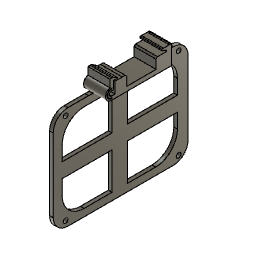
Mounting rack for editing v6 (Autodesk Fusion 360 design; units mm, degrees)
Autodesk Fusion 360 part; units mm, degrees
sketch "Sketch5" plane through (0, 0, 0) normal (1, 0, 0) x (0, 1, 0)
  line L0 (-84.5941, 0) -> (-12.7245, 0)
  line L1 (-2.7245, 10) -> (-2.7245, 59.9846)
  line L2 (-94.5941, 59.9846) -> (-94.5941, 10)
  arc A0 (-9.9546, 50) -> (-24.9546, 65) centre (-24.9546, 50) ccw
  arc A1 (-24.9546, 5) -> (-9.9546, 20) centre (-24.9546, 20) ccw
  arc A2 (-9.9546, 50) -> (-24.9546, 65) centre (-24.9546, 50) ccw
  arc A3 (-73.512, 64.9595) -> (-88.512, 49.9595) centre (-73.512, 49.9595) ccw
  arc A4 (-88.512, 20) -> (-73.512, 5) centre (-73.512, 20) ccw
  line L3 (-88.512, 49.9595) -> (-88.512, 40)
  line L4 (-88.512, 30) -> (-88.512, 20)
  line L5 (-9.9546, 40) -> (-9.9546, 50)
  line L6 (-9.9546, 30) -> (-9.9546, 20)
  arc A5 (-84.5942, 69.9846) -> (-94.5941, 59.9846) centre (-84.5941, 59.9846) ccw
  arc A6 (-94.5941, 10) -> (-84.5941, 0) centre (-84.5941, 10) ccw
  arc A7 (-2.7245, 59.9846) -> (-12.7245, 69.9846) centre (-12.7245, 59.9846) ccw
  arc A8 (-12.7245, 0) -> (-2.7245, 10) centre (-12.7245, 10) ccw
  line L7 (-54.512, 65.0011) -> (-54.512, 40)
  line L8 (-54.512, 5) -> (-54.512, 30)
  line L9 (-43.9546, 5) -> (-43.9546, 30)
  line L10 (-43.9546, 30) -> (-43.9546, 5)
  line L11 (-43.9546, 40) -> (-43.9546, 65)
  line L12 (-43.9546, 65) -> (-24.9546, 65)
  line L13 (-88.512, 40) -> (-54.512, 40)
  line L14 (-43.9546, 40) -> (-9.9546, 40)
  line L15 (-9.9546, 30) -> (-43.9546, 30)
  line L16 (-54.512, 30) -> (-88.512, 30)
  line L17 (-24.9546, 5) -> (-43.9546, 5)
  line L18 (-54.512, 5) -> (-73.512, 5)
  circle A9 centre (-9.125, 65.9) radius 1.6
  circle A10 centre (-86.15, 65.9) radius 1.6
  circle A11 centre (-86.15, 4.1) radius 1.6
  circle A12 centre (-9.125, 4.1) radius 1.6
  line L19 (-12.7245, 69.9846) -> (-26.5, 69.9846)
  line L20 (-70.5614, 69.9846) -> (-84.5942, 69.9846)
  line L21 (-34.0009, 82) -> (-35, 82)
  line L22 (-35, 82) -> (-34.0009, 82)
  line L23 (-27.9827, 84.0115) -> (-28, 84)
  line L24 (-70.5614, 69.9846) -> (-67.5615, 69.9481)
  line L25 (-34.0009, 82) -> (-31, 82)
  line L26 (-37, 75) -> (-37, 81)
  line L27 (-37, 81) -> (-36, 82)
  line L28 (-36, 82) -> (-35, 82)
  line L29 (-60.0004, 81.9976) -> (-65.0026, 81.9977)
  line L30 (-58.0026, 81.9976) -> (-60.0004, 81.9976)
  line L31 (-57.0016, 75) -> (-57.0017, 80.9968)
  line L32 (-57.0017, 80.9968) -> (-58.0026, 81.9976)
  line L33 (-27.9827, 84.9818) -> (-32, 84.9805)
  line L34 (-33.0028, 84.9804) -> (-32, 84.9805)
  line L35 (-27.9827, 84.9818) -> (-27, 84.9823)
  line L36 (-67.5373, 71.9431) -> (-67.5615, 69.9481)
  line L37 (-65.0026, 81.9977) -> (-65.0028, 74.4319)
  line L38 (-66.997, 73.4735) -> (-66.997, 72.9714)
  line L39 (-67, 84.9613) -> (-65.9808, 84.9613)
  line L40 (-65.9808, 84.9613) -> (-63.0198, 82.9885)
  line L41 (-63.0198, 82.9885) -> (-66.0024, 82.9882)
  line L42 (-66.0024, 82.9882) -> (-66.0019, 77.4756)
  line L43 (-66.0019, 77.4756) -> (-67.4929, 77.4715)
  arc A13 (-68.4416, 79.8377) -> (-67.5373, 71.9431) centre (-67.4887, 75.9478) ccw
  arc A14 (-67.01, 78.9263) -> (-66.997, 72.9714) centre (-67.4887, 75.9478) ccw
  arc A15 (-67.01, 78.4247) -> (-66.997, 73.4735) centre (-67.4887, 75.9478) ccw
  arc A16 (-67.4929, 77.4715) -> (-67.4839, 74.4241) centre (-67.4887, 75.9478) ccw
  line L44 (-67.01, 78.4247) -> (-67.01, 78.9263)
  line L45 (-67.4839, 74.4241) -> (-65.0028, 74.4319)
  line L46 (-73.512, 64.9595) -> (-54.512, 65.0011)
  line L47 (-67, 84.9613) -> (-68.458, 84.9566)
  line L48 (-68.458, 84.9566) -> (-68.4416, 79.8377)
  line L49 (-31, 82) -> (-36, 82)
  line L50 (-65.0026, 81.9977) -> (-58.0026, 81.9976)
  line L51 (-57.0016, 75) -> (-37, 75)
  line L52 (-27, 84.9823) -> (-26.5, 84.9823)
  line L53 (-31, 82) -> (-30.0024, 82)
  line L54 (-30.0024, 82) -> (-30.0024, 82.9905)
  line L55 (-30.0024, 82.9905) -> (-30.0024, 82)
  line L56 (-33.0028, 84.9804) -> (-33.0027, 83.9899)
  line L57 (-33.0027, 83.9899) -> (-30.0024, 82.9905)
  line L58 (-26.5, 84.9823) -> (-26.5, 69.9846)
  line L59 (-67.5373, 71.9431) -> (-26.5, 71.9431)
  dimension "d19" = 15
  dimension "d20" = 10
  dimension "d28" = 3.2
  dimension "d31" = 3.2
  dimension "d32" = 3.2
  dimension "d33" = 3.2
  dimension "d63" = 25
  dimension "d64" = 10
  dimension "d65" = 5
  dimension "d169" = 7
  dimension "d181" = 36
  constraint horizontal L0
  constraint vertical L1
  constraint horizontal L19
  constraint vertical L2
  constraint horizontal L17
  constraint tangent A1 L17
  constraint equal A0 A1
  constraint equal A0 A3
  constraint tangent A4 L17
  constraint equal A0 A4
  constraint tangent A3 L3
  constraint tangent A4 L4
  constraint tangent A0 L5
  constraint tangent A1 L6
  constraint tangent A5 L19
  constraint tangent L2 A5
  constraint tangent L0 A6
  constraint tangent L2 A6
  constraint equal A5 A6
  constraint tangent L1 A7
  constraint tangent A7 L19
  constraint equal A5 A7
  constraint tangent L0 A8
  constraint tangent L1 A8
  constraint equal A5 A8
  constraint perpendicular L7 L13
  constraint coincident L8.start L17
  constraint coincident L8.end L15
  constraint perpendicular L8 L15
  constraint perpendicular L9 L17
  constraint coincident L11.start L13
  constraint tangent A2 L12
  constraint collinear L13 L14
  constraint collinear L15 L16
  constraint collinear L17 L18
  constraint coincident L20.start L19
  constraint collinear L19 L20
  constraint horizontal L21
  constraint perpendicular L26 L28
  constraint horizontal L30
  constraint perpendicular L24 L36
  constraint perpendicular L29 L37
  constraint concentric A13 A14
  constraint concentric A14 A15
  constraint concentric A14 A16
  constraint perpendicular L37 L39
  constraint perpendicular L41 L42
  constraint tangent L43 A16
  constraint tangent A16 L45
  constraint perpendicular L47 L48
  constraint perpendicular L26 L51
  constraint parallel L22 L53
  constraint perpendicular L53 L54
  constraint perpendicular L34 L56
  constraint horizontal L52
  constraint perpendicular L19 L58
  constraint coincident L58 L59.end
  constraint perpendicular L58 L59
  measures "d19" radius of A0
  measures "d20" radius of A5
  measures "d28" diameter of A9
  measures "d31" diameter of A10
  measures "d32" diameter of A11
  measures "d33" diameter of A12
  measures "d63" distance of L16 L18
  measures "d64" distance of L13 L16
  measures "d65" distance of L0 L18
  measures "d169" horizontal distance of L29.end L30.start
  measures "d181" distance of L41.end L54.end
extrude "Extrude51" add sketch "Sketch5" along normal blind 2.5 contours L0 L1 L2 A5 A6 A7 A8 L19 L20 L24 L36 L58 L59
extrude "Extrude52" add sketch "Sketch5" along normal blind 15 contours L21 L22 L25 L26 L27 L28 L29 L30 L31 L32 L33 L34 L35 L37 L39 L40 L41 L42 L43 A13 A16 L45 L47 L48 L49 L50 L51 L52 L53 L54 L55 L56 L57 L58 L59
extrude "Extrude47" [rolled back] along distance 15 taper angle 0
extrude "Extrude48" [rolled back] along distance 0.5 taper angle 0
extrude "Extrude49" [rolled back] side1offset 0 taper angle 0
extrude "Extrude50" [rolled back] side1offset 0 taper angle 0
move_body "Move6" [rolled back] rotate angle -90
move_body "Move7" [rolled back]
